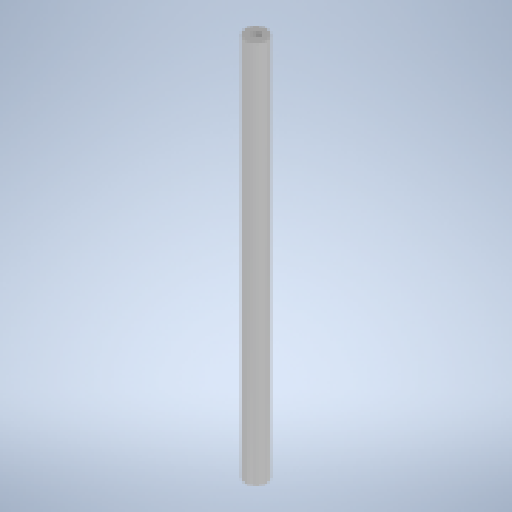
# Autodesk Inventor part: barre
Saved by Autodesk Inventor 2024.2 (Build 282272000, 272)
## iProperties
Created: 2024-09-10
Part Number: barre
Material: Aluminium 6061
Document SubType Name: Modeling
Designer: Sebastien
Density: 2.7 g/cm^3
Appearance: Aluminium - Plat
Author: Sebastien
Autodesk Inventor part; units mm, degrees
ref_plane "YZ Plane" through (0, 0, 0) normal (1, 0, 0) x (0, 1, 0)
ref_plane "XZ Plane" through (0, 0, 0) normal (0, 1, 0) x (-1, 0, 0)
ref_plane "XY Plane" through (0, 0, 0) normal (0, 0, 1) x (1, 0, 0)
sketch "Esquisse1" plane through (0, 0, 0) normal (0, 0, 1) x (1, 0, 0)
  line L0 (0, 0) -> (5, 0)
  line L1 (5, 0) -> (5, 90)
  line L2 (5, 90) -> (0, 90)
  line L3 (0, 90) -> (0, 0)
  dimension "d0" = 10
  dimension "d3" = 180
  constraints: 8 end point, 2 parallel, 1 horizontal, 1 perpendicular
  measures "d0" diameter of L1 L3
  measures "d3" diameter of L2 L0
revolve "Révolution1" add sketch "Esquisse1" angle 360 about axis through (0, 90, 0) along (0, -1, 0)
sketch "Esquisse2" plane through (0, 90, 0) normal (0, 1, 0) x (1, 0, 0)
  circle A0 centre (0, 0) radius 5 projected
  constraints: 1 coincident
hole "Perçage1" at (0, 90, 0) direction (0, -1, 0) diameter 3.242 depth 20 tip angle 118 thread size "M4x0.7" class "6H" standard "ISO Metric profile"
mirror "Mise en miroir1" about plane through (0, 0, 0) normal (0, 1, 0)
